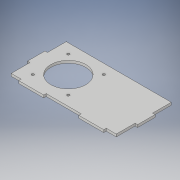
# Autodesk Inventor part: Part Sisi 1
Saved by Autodesk Inventor 2019 (Build 230136000, 136)
## iProperties
Created: 2019-07-08
Part Number: Part Sisi 1
Material: Generic
Document SubType Name: Modeling
Designer: azriel
Density: 1 g/cm^3
Appearance: Default
Author: azriel
Autodesk Inventor part; units mm, degrees
ref_plane "YZ Plane" through (0, 0, 0) normal (1, 0, 0) x (0, 1, 0)
ref_plane "XZ Plane" through (0, 0, 0) normal (0, 1, 0) x (-1, 0, 0)
ref_plane "XY Plane" through (0, 0, 0) normal (0, 0, 1) x (1, 0, 0)
sketch "Sketch1" plane through (0, 0, 0) normal (0, 1, 0) x (-1, 0, 0)
  line L0 (4.6863, 62.0394) -> (4.6863, 67.0394)
  line L1 (4.6863, 67.0394) -> (54.6863, 67.0394)
  line L2 (54.6863, 67.0394) -> (54.6863, 62.0394)
  line L3 (74.6863, 62.0394) -> (54.6863, 62.0394)
  line L4 (-65.3137, 62.0394) -> (-65.3137, 67.0394)
  line L5 (-65.3137, 67.0394) -> (-115.3137, 67.0394)
  line L6 (-115.3137, 67.0394) -> (-115.3137, 62.0394)
  line L7 (4.6863, 62.0394) -> (-65.3137, 62.0394)
  line L8 (-115.3137, 62.0394) -> (-135.3137, 62.0394)
  circle A0 centre (15.4931, 7.0394) radius 35
  line L9 (-135.3137, -47.9606) -> (-115.3137, -47.9606)
  line L10 (-65.3137, -47.9606) -> (4.6863, -47.9606)
  line L11 (54.6863, -47.9606) -> (74.6863, -47.9606)
  line L12 (79.6863, -10.4606) -> (74.6863, -10.4606)
  line L13 (74.6863, -10.4606) -> (74.6863, -47.9606)
  line L14 (79.6863, -10.4606) -> (79.6863, 24.5394)
  line L15 (79.6863, 24.5394) -> (74.6863, 24.5394)
  line L16 (74.6863, 24.5394) -> (74.6863, 62.0394)
  line L17 (-140.3137, -10.4606) -> (-140.3137, 24.5394)
  line L18 (-140.3137, -10.4606) -> (-135.3137, -10.4606)
  line L19 (-135.3137, -10.4606) -> (-135.3137, -47.9606)
  line L20 (-140.3137, 24.5394) -> (-135.3137, 24.5394)
  line L21 (-135.3137, 24.5394) -> (-135.3137, 62.0394)
  line L22 (-115.3137, -47.9606) -> (54.6863, -47.9606)
  circle A1 centre (50.9931, -28.4606) radius 2.5
  circle A2 centre (-20.0069, -28.4606) radius 2.5
  circle A3 centre (-20.0069, 42.5394) radius 2.5
  circle A4 centre (50.9931, 42.5394) radius 2.5
  point P0 (0, 0)
  dimension "d6" = 50
  dimension "d7" = 5
  dimension "d9" = 50
  dimension "d10" = 5
  dimension "d12" = 70
  dimension "d13" = 50
  dimension "d29" = 70
  dimension "d44" = 5
  dimension "d45" = 5
  dimension "d46" = 5
  dimension "d47" = 5
  constraints: 46 end point, 11 parallel, 5 centre point, 5 perpendicular, 3 horizontal, 2 point on line, 1 vertical
  measures "d6" distance of L2.end L0.start
  measures "d7" distance of L0.start L0.end
  measures "d9" distance of L6.end L4.start
  measures "d10" distance of L4.end L4.start
  measures "d12" distance between parallel lines of L4 L0
  measures "d13" distance between parallel lines of L0 L2
  measures "d29" diameter of A0
  measures "d44" diameter of A1
  measures "d45" diameter of A2
  measures "d46" diameter of A3
  measures "d47" diameter of A4
extrude "Extrusion3" add sketch "Sketch1" along normal blind 5
body "Solid3"
